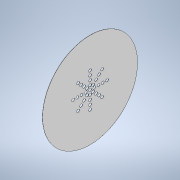
# Autodesk Inventor part: Fan_cover_flat
Saved by Autodesk Inventor 2021 (Build 250183000, 183)
## iProperties
Created: 2021-07-07
Part Number: Fan_cover_flat
Material: Generic
Document SubType Name: Sheet Metal
Designer: MOGIRE
Density: 1 g/cm^3
Appearance: Default
Sheet Metal Rule: Default_mm
Author: MOGIRE
Autodesk Inventor part; units mm, degrees
ref_plane "YZ Plane" through (0, 0, 0) normal (1, 0, 0) x (0, 1, 0)
ref_plane "XZ Plane" through (0, 0, 0) normal (0, 1, 0) x (-1, 0, 0)
ref_plane "XY Plane" through (0, 0, 0) normal (0, 0, 1) x (1, 0, 0)
sketch "Sketch1" plane through (0, 0, 0) normal (1, 0, 0) x (0, 1, 0)
  circle A0 centre (0, 0) radius 210 construction
  line L0 (0, 0) -> (210, 0) construction
  circle A1 centre (0, 0) radius 210
  line L1 (0, 0) -> (148.4924, 148.4924) construction
  line L2 (0, 0) -> (0, 210) construction
  circle A2 centre (0, 0) radius 12.5
  circle A3 centre (37.5, 0) radius 12.5
  circle A4 centre (75, 0) radius 12.5
  circle A5 centre (112.5, 0) radius 12.5
  circle A6 centre (150, 0) radius 12.5
  circle A7 centre (0, 37.5) radius 12.5
  circle A8 centre (0, 75) radius 12.5
  circle A9 centre (0, 112.5) radius 12.5
  circle A10 centre (0, 150) radius 12.5
  circle A11 centre (0, -37.5) radius 12.5
  circle A12 centre (0, -75) radius 12.5
  circle A13 centre (0, -112.5) radius 12.5
  circle A14 centre (0, -150) radius 12.5
  circle A15 centre (-37.5, 0) radius 12.5
  circle A16 centre (-75, 0) radius 12.5
  circle A17 centre (-112.5, 0) radius 12.5
  circle A18 centre (-150, 0) radius 12.5
  circle A19 centre (26.5165, 26.5165) radius 12.5
  circle A20 centre (53.033, 53.033) radius 12.5
  circle A21 centre (79.5495, 79.5495) radius 12.5
  circle A22 centre (106.066, 106.066) radius 12.5
  circle A23 centre (-26.5165, 26.5165) radius 12.5
  circle A24 centre (-53.033, 53.033) radius 12.5
  circle A25 centre (-79.5495, 79.5495) radius 12.5
  circle A26 centre (-106.066, 106.066) radius 12.5
  circle A27 centre (-53.033, -53.033) radius 12.5
  circle A28 centre (-79.5495, -79.5495) radius 12.5
  circle A29 centre (-106.066, -106.066) radius 12.5
  circle A30 centre (-26.5165, -26.5165) radius 12.5
  circle A31 centre (26.5165, -26.5165) radius 12.5
  circle A32 centre (53.033, -53.033) radius 12.5
  circle A33 centre (79.5495, -79.5495) radius 12.5
  circle A34 centre (106.066, -106.066) radius 12.5
  circle A35 centre (0, 0) radius 419.437
  dimension "d0" = 420
  dimension "d1" = 210
  dimension "d2" = 45
  dimension "d3" = 25
  dimension "d4" = 25
  dimension "d5" = 25
  dimension "d6" = 25
  dimension "d7" = 25
  dimension "d8" = 37.5
  dimension "d9" = 37.5
  dimension "d10" = 37.5
  dimension "d11" = 37.5
  dimension "d12" = 25
  dimension "d13" = 25
  dimension "d14" = 25
  dimension "d15" = 25
  dimension "d16" = 37.5
  dimension "d17" = 37.5
  dimension "d18" = 37.5
  dimension "d19" = 37.5
  dimension "d20" = 209.437
  measures "d0" diameter of A0
  measures "d1" distance of L0.start L1.end
  measures "d2" angle of L0 L1
  measures "d3" diameter of A2
  measures "d4" diameter of A3
  measures "d5" diameter of A4
  measures "d6" diameter of A5
  measures "d7" diameter of A6
  measures "d8" distance of A3.centre L0.start
  measures "d9" distance of A4.centre A3.centre
  measures "d10" distance of A5.centre A4.centre
  measures "d11" distance of A6.centre A5.centre
  measures "d12" diameter of A19
  measures "d13" diameter of A20
  measures "d14" diameter of A21
  measures "d15" diameter of A22
  measures "d16" distance of A19.centre L0.start
  measures "d17" distance of A20.centre A19.centre
  measures "d18" distance of A21.centre A20.centre
  measures "d19" distance of A22.centre A21.centre
  measures "d20" radial gap between concentric circles of A35 A0
extrude "Plate1" add sketch "Sketch1" along normal blind 1.5 contours A1 | A35
equation "\"d9\" = d8"
equation "\"d10\" = d9"
equation "\"d11\" = d10"
equation "\"d16\" = d11"
equation "\"d17\" = d11"
equation "\"d18\" = d11"
equation "\"d21\" = Thickness"
equation "\"BendRadius\" = Thickness"
equation "\"BendReliefWidth\" = Thickness"
equation "\"BendReliefDepth\" = 0.5 * Thickness"
equation "\"CornerReliefSize\" = 4 * Thickness"
equation "\"MinimumRemnant\" = 2 * Thickness"
equation "\"TransitionRadius\" = BendRadius"
equation "\"JacobiRadiusSize\" = BendRadius"
equation "\"GapSize\" = Thickness"
equation "\"Thickness\" = 1.5"
body "Solid1"
